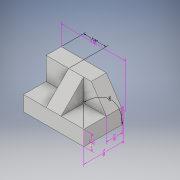
# Autodesk Inventor part: Part3
Saved by Autodesk Inventor 2018 (Build 220112000, 112)
## iProperties
Created: 2018-11-28
Part Number: Part3
Material: Generic
Document SubType Name: Modeling
Designer: 10043883
Density: 1 g/cm^3
Appearance: Default
Author: 10043883
Autodesk Inventor part; units mm, degrees
ref_plane "YZ Plane" through (0, 0, 0) normal (1, 0, 0) x (0, 1, 0)
ref_plane "XZ Plane" through (0, 0, 0) normal (0, 1, 0) x (-1, 0, 0)
ref_plane "XY Plane" through (0, 0, 0) normal (0, 0, 1) x (1, 0, 0)
sketch "Sketch1" plane through (0, 0, 0) normal (0, 1, 0) x (-1, 0, 0)
  line L0 (0, 0) -> (203.2, 0)
  line L1 (203.2, 0) -> (203.2, -127)
  line L2 (203.2, -127) -> (0, -127)
  line L3 (0, -127) -> (0, 0)
  dimension "d0" = 203.2
  dimension "d1" = 127
  constraints: 8 end point, 2 parallel, 1 horizontal, 1 perpendicular
  measures "d0" distance of L1.end L2.end
  measures "d1" distance of L0.end L1.end
extrude "Extrusion1" add sketch "Sketch1" along normal blind 50.8
sketch "Sketch2" plane through (0, 50.8, 0) normal (0, 1, 0) x (1, 0, 0)
  line L0 (-203.2, 127) -> (-203.2, 0) projected
  line L1 (-203.2, 76.2) -> (0, 76.2)
  line L2 (0, 76.2) -> (0, 127)
  line L3 (0, 127) -> (-203.2, 127)
  line L4 (-203.2, 127) -> (-203.2, 76.2)
  point P0 (0, 0)
  dimension "d4" = 50.8
  dimension "d13" = 203.2
  constraints: 8 end point, 2 parallel, 1 horizontal, 1 perpendicular, 1 point on line
  measures "d4" distance of L2.end L1.end
  measures "d13" distance of L3.end L2.end
extrude "Extrusion2" add sketch "Sketch2" along normal blind 76.2
chamfer "Chamfer1" distance 50.8 angle 56.31 1 edges at (0, 127, -101.6) measured on face at (-67.7333, 127, -110.0667)
sketch "Sketch3" plane through (0, 50.8, 0) normal (0, 1, 0) x (1, 0, 0)
  line L0 (0, 76.2) -> (-203.2, 76.2) projected
  line L1 (-127, 76.2) -> (-76.2, 76.2)
  line L2 (-76.2, 76.2) -> (-76.2, 0)
  line L3 (-76.2, 0) -> (-127, 0)
  line L4 (-127, 0) -> (-127, 76.2)
  line L5 (-203.2, 76.2) -> (-203.2, 0) projected
  point P0 (0, 0)
  dimension "d10" = 50.8
  dimension "d11" = 76.2
  dimension "d12" = 76.2
  constraints: 8 end point, 2 parallel, 1 horizontal, 1 perpendicular, 1 point on line
  measures "d10" distance of L2.end L3.end
  measures "d11" distance of L1.end L2.end
  measures "d12" distance from line of L5 L3.end
extrude "Extrusion3" add sketch "Sketch3" along normal blind 76.2
chamfer "Chamfer2" distance 76.2 angle 45 1 edges at (-101.6, 127, 0)
sketch "Sketch4" plane through (-0.0002, 50.7998, -127) normal (0.8321, 0.5547, 0) x (-0.5547, 0.8321, 0)
  point P0 (-42.2682, 127)
sketch "Sketch5" plane through (0, 127, 0) normal (0, 1, 0) x (1, 0, 0)
  point P0 (0, 0)
sketch "Sketch6" plane through (-50.8, 127, -127) normal (0.8321, 0.5547, 0) x (-0.5547, 0.8321, 0)
  point P0 (-133.8492, 127)
body "Solid1"
